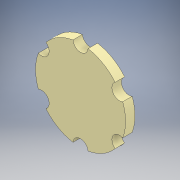
# Autodesk Inventor part: led
Saved by Autodesk Inventor 2017 (Build 210142000, 142)
## iProperties
Created: 2018-04-04
Part Number: led
Material: Generic
Document SubType Name: Modeling
Designer: dasae
Density: 1 g/cm^3
Appearance: Default
Author: dasae
Autodesk Inventor part; units mm, degrees
ref_plane "YZ Plane" through (0, 0, 0) normal (1, 0, 0) x (0, 1, 0)
ref_plane "XZ Plane" through (0, 0, 0) normal (0, 1, 0) x (-1, 0, 0)
ref_plane "XY Plane" through (0, 0, 0) normal (0, 0, 1) x (1, 0, 0)
sketch "Sketch1" plane through (0, 0, 0) normal (0, 1, 0) x (-1, 0, 0)
  arc A0 (1.5943, -9.3653) -> (-1.5943, -9.3653) centre (0, -9.5) ccw
  arc A1 (8.9077, -3.3019) -> (7.3134, -6.0634) centre (8.2272, -4.75) ccw
  arc A2 (7.3134, 6.0634) -> (8.9077, 3.3019) centre (8.2272, 4.75) ccw
  arc A3 (-1.5943, 9.3653) -> (1.5943, 9.3653) centre (0, 9.5) ccw
  arc A4 (-8.9077, 3.3019) -> (-7.3134, 6.0634) centre (-8.2272, 4.75) ccw
  arc A5 (-7.3134, -6.0634) -> (-8.9077, -3.3019) centre (-8.2272, -4.75) ccw
  arc A6 (1.5943, -9.3653) -> (7.3134, -6.0634) centre (0, 0) ccw
  arc A7 (8.9077, -3.3019) -> (8.9077, 3.3019) centre (0, 0) ccw
  arc A8 (7.3134, 6.0634) -> (1.5943, 9.3653) centre (0, 0) ccw
  arc A9 (-1.5943, 9.3653) -> (-7.3134, 6.0634) centre (0, 0) ccw
  arc A10 (-8.9077, 3.3019) -> (-8.9077, -3.3019) centre (0, 0) ccw
  arc A11 (-7.3134, -6.0634) -> (-1.5943, -9.3653) centre (0, 0) ccw
  dimension "d1" = 3.2
  dimension "d4" = 360
  constraints: 24 point on circle, 12 centre point, 1 coincident, 25 other
  measures "d1" diameter of A0
extrude "Extrusion1" add sketch "Sketch1" along normal blind 2
sketch "Sketch2" plane through (0, 2, 0) normal (0, 1, 0) x (1, 0, 0)
  line L0 (2, 2) -> (-2, 2)
  line L1 (-2, 2) -> (-2, -2)
  line L2 (-2, -2) -> (2, -2)
  line L3 (2, -2) -> (2, 2)
  line L4 (2, 2) -> (-2, -2) construction
  line L5 (-2, 2) -> (2, -2) construction
  point P0 (0, 0)
  dimension "d8" = 4
  dimension "d9" = 4
  constraints: 12 end point, 2 midpoint, 2 parallel, 1 horizontal, 1 perpendicular
  measures "d8" distance of L2.end L1.end
  measures "d9" distance of L1.end L0.end
extrude "Extrusion2" add sketch "Sketch2" along normal blind 2
body "Solid1"
